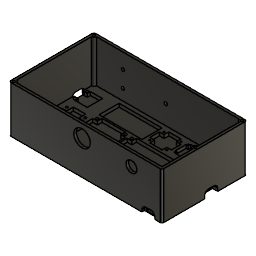
Base TestBenchV2 v1 (Autodesk Fusion 360 design; units mm, degrees)
part number: 2025-10-03-12-35-34-740
Autodesk Fusion 360 part; units mm, degrees
(part 1 of 3)
sketch "Boceto4" plane through (0, 0, 0) normal (0, 0, 1) x (1, 0, 0)
  line L0 (165, 0) -> (165, 100)
  line L1 (165, 0) -> (0, 0)
  line L2 (165, 100) -> (0, 100)
  line L3 (0, 100) -> (0, 0)
  line L4 (0, 100) -> (-15, 100)
  line L5 (-15, 100) -> (-15, 0)
  line L6 (-15, 0) -> (0, 0)
  line L7 (0, 0) -> (0, 100)
  dimension "d157" = 165
  dimension "d168" = 100
  dimension "d277" = 15
  constraint vertical L0
  constraint perpendicular L0 L1
  constraint perpendicular L0 L2
  constraint coincident L1.end L3.end
  constraint horizontal L4
  constraint vertical L5
  constraint horizontal L6
  constraint vertical L7
  constraint collinear L1 L6
  measures "d157" distance of L0.start L1.end
  measures "d168" distance of L1 L2
  measures "d277" distance of L2.end L4.end
extrude "Extruir2" add sketch "Boceto4" along normal blind 5
sketch "Boceto1" plane through (0, 0, 5) normal (0, 0, 1) x (1, 0, 0)
  line L0 (22, 67) -> (60.5, 67)
  line L1 (60.5, 67) -> (60.5, 16.5)
  line L2 (60.5, 16.5) -> (22, 16.5)
  line L3 (22, 16.5) -> (22, 67)
  line L4 (62.5, 67) -> (137.5, 67)
  line L5 (137.5, 67) -> (137.5, 16.5)
  line L6 (137.5, 16.5) -> (62.5, 16.5)
  line L7 (62.5, 16.5) -> (62.5, 67)
  line L8 (103.5, 92.5293) -> (147, 92.5293)
  line L9 (147, 74.5293) -> (103.5, 74.5293)
  line L10 (103.5, 74.5293) -> (103.5, 92.5293)
  line L11 (75, 92.5) -> (100.5, 92.5)
  line L12 (100.5, 92.5) -> (100.5, 70.2)
  line L13 (100.5, 70.2) -> (75, 70.2)
  line L14 (75, 70.2) -> (75, 92.5)
  line L15 (165, 0) -> (165, 100)
  line L16 (165, 100) -> (-15, 100)
  line L17 (-15, 0) -> (165, 0)
  line L18 (22, 92.5) -> (72.5, 92.5)
  line L19 (72.5, 92.5) -> (72.5, 69)
  line L20 (72.5, 69) -> (22, 69)
  line L21 (22, 69) -> (22, 92.5)
  line L22 (-10.5, 87.487) -> (7.5, 87.487)
  line L23 (7.5, 87.487) -> (7.5, 69.487)
  line L24 (7.5, 69.487) -> (-10.5, 69.487)
  line L25 (-7.0254, 61.685) -> (19.3746, 61.685)
  line L26 (19.3746, 61.685) -> (19.3746, 24.785)
  line L27 (19.3746, 24.785) -> (-7.0254, 24.785)
  line L28 (-7.0254, 24.785) -> (-7.0254, 61.685)
  line L29 (139.5, 49) -> (139.5, 67)
  line L30 (157.5, 49) -> (139.5, 49)
  line L31 (139.5, 67) -> (157.5, 67)
  line L32 (140, 4.5) -> (140, 22.5)
  line L33 (140, 22.5) -> (158, 22.5)
  line L34 (158, 22.5) -> (158, 4.5)
  line L35 (-10.5, 73.487) -> (-12, 73.487)
  line L36 (-12, 83.487) -> (-12, 73.487)
  line L37 (-10.5, 69.487) -> (-10.5, 73.487)
  line L38 (-10.5, 83.487) -> (-10.5, 87.487)
  line L39 (144, 3) -> (144, 4.5)
  line L40 (154, 3) -> (154, 4.5)
  line L41 (158, 4.5) -> (154, 4.5)
  line L42 (144, 4.5) -> (140, 4.5)
  line L43 (159, 63) -> (157.5, 63)
  line L44 (157.5, 53) -> (159, 53)
  line L45 (165, 63) -> (165, 53)
  line L46 (157.5, 67) -> (157.5, 63)
  line L47 (157.5, 53) -> (157.5, 49)
  circle A0 centre (-12, 97) radius 1.5
  circle A1 centre (162, 97) radius 1.5
  circle A2 centre (-12, 3) radius 1.5
  circle A3 centre (162, 42) radius 1.5
  line L48 (147, 89.5293) -> (165, 89.5293)
  line L49 (147, 77.5293) -> (165, 77.5293)
  line L50 (147, 92.5293) -> (147, 89.5293)
  line L51 (147, 77.5293) -> (147, 74.5293)
  line L52 (165, 89.5293) -> (165, 77.5293)
  line L53 (112.793, 73.7793) -> (132.793, 73.7793)
  line L54 (132.793, 73.7793) -> (132.793, 67.7793)
  line L55 (132.793, 67.7793) -> (112.793, 67.7793)
  line L56 (112.793, 67.7793) -> (112.793, 73.7793)
  line L57 (-15, 100) -> (-15, 0)
  line L58 (154, 3) -> (144, 3)
  line L59 (-12, 83.487) -> (-10.5, 83.487)
  line L60 (159, 63) -> (159, 53)
  dimension "d7" = 38.5
  dimension "d8" = 50.5
  dimension "d9" = 75
  dimension "d10" = 50.5
  dimension "d17" = 43.5
  dimension "d18" = 18
  dimension "d21" = 25.5
  dimension "d22" = 22.3
  dimension "d160" = 50.5
  dimension "d161" = 23.5
  dimension "d162" = 18
  dimension "d163" = 18
  dimension "d164" = 26.4
  dimension "d165" = 36.9
  dimension "d169" = 18
  dimension "d170" = 18
  dimension "d171" = 18
  dimension "d172" = 18
  dimension "d174" = 4
  dimension "d175" = 4
  dimension "d176" = 4
  dimension "d177" = 4
  dimension "d179" = 4
  dimension "d180" = 3
  dimension "d181" = 3
  dimension "d183" = 3
  dimension "d184" = 3
  dimension "d185" = 3
  dimension "d186" = 3
  dimension "d187" = 3
  dimension "d189" = 3
  dimension "d190" = 3
  dimension "d191" = 7
  dimension "d194" = 3
  dimension "d195" = 3
  dimension "d266" = 20
  dimension "d267" = 6
  dimension "d268" = 0.75
  dimension "d278" = 3
  dimension "d279" = 3
  dimension "d280" = 1.5
  dimension "d310" = 3
  dimension "d311" = 1.5
  dimension "d312" = 3
  dimension "d313" = 1.5
  constraint horizontal L0
  constraint vertical L1
  constraint horizontal L2
  constraint vertical L3
  constraint horizontal L4
  constraint vertical L5
  constraint horizontal L6
  constraint vertical L7
  constraint horizontal L8
  constraint vertical L50
  constraint horizontal L9
  constraint vertical L10
  constraint horizontal L11
  constraint vertical L12
  constraint horizontal L13
  constraint vertical L14
  constraint horizontal L18
  constraint vertical L19
  constraint horizontal L20
  constraint vertical L21
  constraint horizontal L22
  constraint vertical L23
  constraint horizontal L24
  constraint vertical L37
  constraint horizontal L25
  constraint vertical L26
  constraint horizontal L27
  constraint vertical L28
  constraint horizontal L31
  constraint vertical L46
  constraint horizontal L30
  constraint vertical L29
  constraint horizontal L33
  constraint vertical L34
  constraint horizontal L41
  constraint vertical L32
  constraint coincident L38.start L37
  constraint collinear L37 L38
  constraint coincident L39.end L41
  constraint perpendicular L39 L41
  constraint perpendicular L40 L41
  constraint collinear L41 L42
  constraint coincident L15 L45.start
  constraint perpendicular L43 L46
  constraint coincident L44.start L46
  constraint coincident L15 L45.end
  constraint perpendicular L15 L44
  constraint collinear L46 L47
  constraint coincident L15 L48.end
  constraint perpendicular L15 L48
  constraint coincident L49.start L50
  constraint coincident L15 L49.end
  constraint perpendicular L15 L49
  constraint collinear L50 L51
  constraint horizontal L53
  constraint vertical L54
  constraint horizontal L55
  constraint vertical L56
  constraint horizontal L58
  constraint perpendicular L38 L59
  constraint vertical L60
  measures "d7" distance of L0.start L0.end
  measures "d8" distance of L0.start L2.end
  measures "d9" distance of L4.start L4.end
  measures "d10" distance of L4.start L6.end
  measures "d17" distance of L8.start L8.end
  measures "d18" distance of L8.start L9.end
  measures "d21" distance of L11.start L11.end
  measures "d22" distance of L11.start L13.end
  measures "d160" distance of L18.start L18.end
  measures "d161" distance of L18.start L20.end
  measures "d162" distance of L22.start L22.end
  measures "d163" distance of L22.start L24.end
  measures "d164" distance of L25.start L25.end
  measures "d165" distance of L25.start L27.end
  measures "d169" distance of L31.end L29.end
  measures "d170" distance of L29.start L29.end
  measures "d171" distance of L32.end L33.end
  measures "d172" distance of L32.end L32.start
  measures "d174" distance of L24 L35
  measures "d175" distance of L34 L40
  measures "d176" distance of L32 L39
  measures "d177" distance of L31 L43
  measures "d179" distance of L30 L44
  measures "d180" diameter of A0
  measures "d181" distance of L16 A0.centre
  measures "d183" diameter of A1
  measures "d184" distance of L15 A1.centre
  measures "d185" distance of L16 A1.centre
  measures "d186" diameter of A2
  measures "d187" distance of L17 A2.centre
  measures "d189" diameter of A3
  measures "d190" distance of L15 A3.centre
  measures "d191" distance of L30 A3.centre
  measures "d194" distance of L8 L48
  measures "d195" distance of L9 L49
  measures "d266" distance of L53.start L53.end
  measures "d267" distance of L53.start L55.end
  measures "d268" distance of L9 L53
  measures "d278" horizontal distance of A2.centre L17.start
  measures "d279" distance of A0.centre L57
  measures "d280" distance of L36 L38
  measures "d310" distance of L36 L57
  measures "d311" distance of L40.start L40.end
  measures "d312" distance of L17 L58
  measures "d313" distance of L43.end L43.start
extrude "Extruir3" cut sketch "Boceto1" against normal blind 4 contours L0 L1 L2 L3 | L4 L5 L6 L7 | L8 L9 L10 L15 L48 L49 L50 L51 L52 | L11 L12 L13 L14 | L18 L19 L20 L21 | L22 L23 L24 L35 L36 L37 L38 L59 | L25 L26 L27 L28 | L29 L30 L31 L43 L44 L46 L47 L60 | L32 L33 L34 L39 L40 L41 L42 L58 | A0 | A1 | A2 | A3 | L53 L54 L55 L56
sketch "Boceto15" plane through (0, 0, 1) normal (0, 0, 1) x (-1, 0, 0)
  line L0 (-140.5294, -30.8793) -> (-140.5328, -29.1153)
  line L1 (-140.5328, -29.1153) -> (-140.2681, -29.1148)
  line L2 (-140.2681, -29.1148) -> (-140.2648, -30.8788)
  line L3 (-140.2648, -30.8788) -> (-139.6058, -30.8776)
  line L4 (-139.6058, -30.8776) -> (-139.6054, -31.1136)
  line L5 (-139.6054, -31.1136) -> (-141.1906, -31.1166)
  line L6 (-141.1906, -31.1166) -> (-141.1911, -30.8806)
  line L7 (-141.1911, -30.8806) -> (-140.5294, -30.8793)
  spline S0 degree 3 poles (-143.6617, -29.1663) (-143.604, -29.1955) (-143.4902, -29.2532) (-143.412, -29.3541) (-143.3734, -29.4038) knots 0 0 0 0 0.019136 0.037772 0.037772 0.037772 0.037772
  spline S1 degree 3 poles (-143.3734, -29.4038) (-143.3426, -29.4589) (-143.2802, -29.5708) (-143.2687, -29.6984) (-143.2629, -29.7631) knots 0 0 0 0 0.018713 0.037965 0.037965 0.037965 0.037965
  line L8 (-143.2629, -29.7631) -> (-143.5125, -29.7854)
  spline S2 degree 3 poles (-143.5125, -29.7854) (-143.5197, -29.7389) (-143.533, -29.6519) (-143.5757, -29.5751) (-143.5955, -29.5393) knots 0 0 0 0 0.013975 0.026155 0.026155 0.026155 0.026155
  spline S3 degree 3 poles (-143.5955, -29.5393) (-143.6215, -29.5083) (-143.6771, -29.4418) (-143.7554, -29.4042) (-143.797, -29.3842) knots 0 0 0 0 0.012002 0.025694 0.025694 0.025694 0.025694
  spline S4 degree 3 poles (-143.797, -29.3842) (-143.8449, -29.3669) (-143.9441, -29.3313) (-144.0496, -29.3274) (-144.1041, -29.3254) knots 0 0 0 0 0.015163 0.031432 0.031432 0.031432 0.031432
  spline S5 degree 3 poles (-144.1041, -29.3254) (-144.152, -29.327) (-144.2433, -29.3299) (-144.3302, -29.3577) (-144.3714, -29.3709) knots 0 0 0 0 0.014301 0.027232 0.027232 0.027232 0.027232
  spline S6 degree 3 poles (-144.3714, -29.3709) (-144.4068, -29.3864) (-144.4732, -29.4155) (-144.5213, -29.4695) (-144.5438, -29.4947) knots 0 0 0 0 0.011435 0.021444 0.021444 0.021444 0.021444
  spline S7 degree 3 poles (-144.5438, -29.4947) (-144.5602, -29.5213) (-144.5928, -29.5739) (-144.5977, -29.6356) (-144.6001, -29.666) knots 0 0 0 0 0.009237 0.018267 0.018267 0.018267 0.018267
  spline S8 degree 3 poles (-144.6001, -29.666) (-144.5979, -29.6962) (-144.5936, -29.7557) (-144.5611, -29.8057) (-144.5452, -29.8303) knots 0 0 0 0 0.008921 0.017573 0.017573 0.017573 0.017573
  spline S9 degree 3 poles (-144.5452, -29.8303) (-144.5221, -29.8534) (-144.4705, -29.9052) (-144.4025, -29.9327) (-144.3649, -29.948) knots 0 0 0 0 0.009698 0.021725 0.021725 0.021725 0.021725
  spline S10 degree 3 poles (-144.3649, -29.948) (-144.3219, -29.9617) (-144.2045, -29.9991) (-144.0846, -30.0271) (-144.0086, -30.0449) knots 0 0 0 0 0.013533 0.036931 0.036931 0.036931 0.036931
  spline S11 degree 3 poles (-144.0086, -30.0449) (-143.9296, -30.0636) (-143.7975, -30.0949) (-143.6725, -30.1477) (-143.6223, -30.169) knots 0 0 0 0 0.024297 0.040637 0.040637 0.040637 0.040637
  spline S12 degree 3 poles (-143.6223, -30.169) (-143.5783, -30.1943) (-143.4947, -30.2423) (-143.4361, -30.3187) (-143.4084, -30.3548) knots 0 0 0 0 0.015064 0.02858 0.02858 0.02858 0.02858
  spline S13 degree 3 poles (-143.4084, -30.3548) (-143.3879, -30.3932) (-143.3462, -30.471) (-143.3406, -30.559) (-143.3377, -30.6036) knots 0 0 0 0 0.012908 0.026139 0.026139 0.026139 0.026139
  spline S14 degree 3 poles (-143.3377, -30.6036) (-143.3413, -30.6535) (-143.3487, -30.7542) (-143.3981, -30.8424) (-143.4231, -30.8869) knots 0 0 0 0 0.014805 0.02991 0.02991 0.02991 0.02991
  spline S15 degree 3 poles (-143.4231, -30.8869) (-143.4559, -30.9285) (-143.5237, -31.0148) (-143.6226, -31.0625) (-143.6738, -31.0872) knots 0 0 0 0 0.01568 0.032466 0.032466 0.032466 0.032466
  spline S16 degree 3 poles (-143.6738, -31.0872) (-143.7313, -31.1072) (-143.8501, -31.1485) (-143.9758, -31.1535) (-144.0406, -31.1561) knots 0 0 0 0 0.018164 0.037509 0.037509 0.037509 0.037509
  spline S17 degree 3 poles (-144.0406, -31.1561) (-144.111, -31.1539) (-144.2454, -31.1496) (-144.3725, -31.106) (-144.433, -31.0852) knots 0 0 0 0 0.021001 0.040071 0.040071 0.040071 0.040071
  spline S18 degree 3 poles (-144.433, -31.0852) (-144.4859, -31.0593) (-144.589, -31.0088) (-144.6601, -30.9188) (-144.6946, -30.8749) knots 0 0 0 0 0.017437 0.033952 0.033952 0.033952 0.033952
  spline S19 degree 3 poles (-144.6946, -30.8749) (-144.7217, -30.8267) (-144.7766, -30.7286) (-144.7878, -30.6168) (-144.7935, -30.56) knots 0 0 0 0 0.016416 0.033327 0.033327 0.033327 0.033327
  line L9 (-144.7935, -30.56) -> (-144.5397, -30.5404)
  spline S20 degree 3 poles (-144.5397, -30.5404) (-144.5301, -30.5986) (-144.5119, -30.7081) (-144.4362, -30.7888) (-144.4007, -30.8266) knots 0 0 0 0 0.017238 0.032462 0.032462 0.032462 0.032462
  spline S21 degree 3 poles (-144.4007, -30.8266) (-144.3531, -30.8547) (-144.2461, -30.9179) (-144.1213, -30.9211) (-144.052, -30.9228) knots 0 0 0 0 0.016321 0.036707 0.036707 0.036707 0.036707
  spline S22 degree 3 poles (-144.052, -30.9228) (-143.9811, -30.9216) (-143.8568, -30.9195) (-143.7486, -30.8598) (-143.7022, -30.8342) knots 0 0 0 0 0.02087 0.036564 0.036564 0.036564 0.036564
  spline S23 degree 3 poles (-143.7022, -30.8342) (-143.6702, -30.8041) (-143.6086, -30.746) (-143.5979, -30.6622) (-143.5928, -30.6218) knots 0 0 0 0 0.012728 0.024562 0.024562 0.024562 0.024562
  spline S24 degree 3 poles (-143.5928, -30.6218) (-143.596, -30.5876) (-143.6023, -30.5198) (-143.6482, -30.4695) (-143.6709, -30.4446) knots 0 0 0 0 0.010013 0.019843 0.019843 0.019843 0.019843
  spline S25 degree 3 poles (-143.6709, -30.4446) (-143.7162, -30.4195) (-143.8409, -30.3503) (-143.981, -30.3213) (-144.0702, -30.3028) knots 0 0 0 0 0.01549 0.042576 0.042576 0.042576 0.042576
  spline S26 degree 3 poles (-144.0702, -30.3028) (-144.1616, -30.2826) (-144.3119, -30.2493) (-144.4565, -30.1967) (-144.5131, -30.1761) knots 0 0 0 0 0.028046 0.046113 0.046113 0.046113 0.046113
  spline S27 degree 3 poles (-144.5131, -30.1761) (-144.5665, -30.1491) (-144.6665, -30.0986) (-144.738, -30.0127) (-144.7714, -29.9726) knots 0 0 0 0 0.017709 0.033187 0.033187 0.033187 0.033187
  spline S28 degree 3 poles (-144.7714, -29.9726) (-144.7957, -29.9294) (-144.8455, -29.8412) (-144.8519, -29.74) (-144.8551, -29.6883) knots 0 0 0 0 0.014678 0.02998 0.02998 0.02998 0.02998
  spline S29 degree 3 poles (-144.8551, -29.6883) (-144.8512, -29.6356) (-144.8433, -29.5286) (-144.7909, -29.4349) (-144.7643, -29.3874) knots 0 0 0 0 0.015669 0.031781 0.031781 0.031781 0.031781
  spline S30 degree 3 poles (-144.7643, -29.3874) (-144.7298, -29.3425) (-144.6586, -29.2499) (-144.5553, -29.1953) (-144.5021, -29.1672) knots 0 0 0 0 0.016779 0.034595 0.034595 0.034595 0.034595
  spline S31 degree 3 poles (-144.5021, -29.1672) (-144.4422, -29.1442) (-144.3182, -29.0967) (-144.1854, -29.091) (-144.1168, -29.088) knots 0 0 0 0 0.019123 0.039562 0.039562 0.039562 0.039562
  spline S32 degree 3 poles (-144.1168, -29.088) (-144.0329, -29.09) (-143.8771, -29.0937) (-143.7297, -29.1434) (-143.6617, -29.1663) knots 0 0 0 0 0.025027 0.046416 0.046416 0.046416 0.046416
  spline S33 degree 3 poles (-148.0234, -29.163) (-147.9747, -29.1532) (-147.8683, -29.1317) (-147.7597, -29.1299) (-147.7008, -29.1289) knots 0 0 0 0 0.014862 0.032497 0.032497 0.032497 0.032497
  line L10 (-147.7008, -29.1289) -> (-146.9382, -29.1275)
  line L11 (-146.9382, -29.1275) -> (-146.9344, -31.1275)
  line L12 (-146.9344, -31.1275) -> (-147.6847, -31.1289)
  spline S34 degree 3 poles (-147.6847, -31.1289) (-147.7542, -31.1278) (-147.8799, -31.1257) (-147.9992, -31.0865) (-148.0525, -31.0689) knots 0 0 0 0 0.020707 0.037453 0.037453 0.037453 0.037453
  spline S35 degree 3 poles (-148.0525, -31.0689) (-148.0961, -31.0461) (-148.183, -31.0008) (-148.2409, -30.9217) (-148.2698, -30.8824) knots 0 0 0 0 0.014555 0.028975 0.028975 0.028975 0.028975
  spline S36 degree 3 poles (-148.2698, -30.8824) (-148.2927, -30.8404) (-148.3377, -30.758) (-148.3451, -30.6644) (-148.3487, -30.6186) knots 0 0 0 0 0.014187 0.027818 0.027818 0.027818 0.027818
  spline S37 degree 3 poles (-148.3487, -30.6186) (-148.3458, -30.5763) (-148.3399, -30.4909) (-148.2998, -30.4152) (-148.2796, -30.377) knots 0 0 0 0 0.01257 0.025379 0.025379 0.025379 0.025379
  spline S38 degree 3 poles (-148.2796, -30.377) (-148.2526, -30.3405) (-148.196, -30.2643) (-148.1131, -30.218) (-148.0698, -30.1938) knots 0 0 0 0 0.013451 0.028132 0.028132 0.028132 0.028132
  spline S39 degree 3 poles (-148.0698, -30.1938) (-148.1261, -30.174) (-148.2339, -30.1361) (-148.3119, -30.0527) (-148.3492, -30.0129) knots 0 0 0 0 0.017587 0.033722 0.033722 0.033722 0.033722
  spline S40 degree 3 poles (-148.3492, -30.0129) (-148.3777, -29.9676) (-148.436, -29.8751) (-148.4435, -29.766) (-148.4473, -29.7102) knots 0 0 0 0 0.015782 0.032266 0.032266 0.032266 0.032266
  spline S41 degree 3 poles (-148.4473, -29.7102) (-148.445, -29.6644) (-148.4405, -29.5738) (-148.4057, -29.4902) (-148.3884, -29.4488) knots 0 0 0 0 0.013638 0.026971 0.026971 0.026971 0.026971
  spline S42 degree 3 poles (-148.3884, -29.4488) (-148.3684, -29.4115) (-148.3305, -29.3407) (-148.2705, -29.2875) (-148.2421, -29.2623) knots 0 0 0 0 0.012583 0.02387 0.02387 0.02387 0.02387
  spline S43 degree 3 poles (-148.2421, -29.2623) (-148.2101, -29.2415) (-148.1423, -29.1974) (-148.0645, -29.1749) (-148.0234, -29.163) knots 0 0 0 0 0.011395 0.024144 0.024144 0.024144 0.024144
  line L13 (-150.9489, -30.7067) -> (-150.9519, -29.1351)
  line L14 (-150.9519, -29.1351) -> (-150.6982, -29.1346)
  line L15 (-150.6982, -29.1346) -> (-150.6944, -31.1346)
  line L16 (-150.6944, -31.1346) -> (-150.9659, -31.1352)
  line L17 (-150.9659, -31.1352) -> (-152.0193, -29.5669)
  line L18 (-152.0193, -29.5669) -> (-152.0163, -31.1371)
  line L19 (-152.0163, -31.1371) -> (-152.2701, -31.1376)
  line L20 (-152.2701, -31.1376) -> (-152.2739, -29.1376)
  line L21 (-152.2739, -29.1376) -> (-152.0024, -29.1371)
  line L22 (-152.0024, -29.1371) -> (-150.9489, -30.7067)
  line L23 (-155.0321, -30.0856) -> (-155.0339, -29.1429)
  line L24 (-155.0339, -29.1429) -> (-154.7692, -29.1424)
  line L25 (-154.7692, -29.1424) -> (-154.7654, -31.1424)
  line L26 (-154.7654, -31.1424) -> (-155.0301, -31.1429)
  line L27 (-155.0301, -31.1429) -> (-155.0316, -30.3216)
  line L28 (-155.0316, -30.3216) -> (-156.0712, -30.3236)
  line L29 (-156.0712, -30.3236) -> (-156.0696, -31.1448)
  line L30 (-156.0696, -31.1448) -> (-156.3343, -31.1453)
  line L31 (-156.3343, -31.1453) -> (-156.3381, -29.1453)
  line L32 (-156.3381, -29.1453) -> (-156.0734, -29.1448)
  line L33 (-156.0734, -29.1448) -> (-156.0716, -30.0875)
  line L34 (-156.0716, -30.0875) -> (-155.0321, -30.0856)
  line L35 (-143.2927, -26.2352) -> (-143.2932, -25.9992)
  line L36 (-143.2932, -25.9992) -> (-141.8007, -25.9963)
  line L37 (-141.8007, -25.9963) -> (-141.7969, -27.9963)
  line L38 (-141.7969, -27.9963) -> (-143.243, -27.9991)
  line L39 (-143.243, -27.9991) -> (-143.2435, -27.763)
  line L40 (-143.2435, -27.763) -> (-142.062, -27.7608)
  line L41 (-142.062, -27.7608) -> (-142.0632, -27.1483)
  line L42 (-142.0632, -27.1483) -> (-143.1696, -27.1504)
  line L43 (-143.1696, -27.1504) -> (-143.17, -26.9157)
  line L44 (-143.17, -26.9157) -> (-142.0636, -26.9136)
  line L45 (-142.0636, -26.9136) -> (-142.0649, -26.2328)
  line L46 (-142.0649, -26.2328) -> (-143.2927, -26.2352)
  spline S44 degree 3 poles (-145.7899, -25.9698) (-145.6994, -25.9773) (-145.5229, -25.9921) (-145.3967, -26.1159) (-145.3353, -26.1763) knots 0 0 0 0 0.026334 0.051363 0.051363 0.051363 0.051363
  spline S45 degree 3 poles (-145.3353, -26.1763) (-145.2777, -26.2834) (-145.1422, -26.5356) (-145.1382, -26.8234) (-145.1359, -26.989) knots 0 0 0 0 0.036009 0.08476 0.08476 0.08476 0.08476
  spline S46 degree 3 poles (-145.1359, -26.989) (-145.1371, -27.0963) (-145.1394, -27.2896) (-145.1867, -27.4768) (-145.2078, -27.5601) knots 0 0 0 0 0.032061 0.057736 0.057736 0.057736 0.057736
  spline S47 degree 3 poles (-145.2078, -27.5601) (-145.2335, -27.6269) (-145.2823, -27.7536) (-145.3786, -27.849) (-145.4241, -27.8941) knots 0 0 0 0 0.021191 0.040192 0.040192 0.040192 0.040192
  spline S48 degree 3 poles (-145.4241, -27.8941) (-145.4766, -27.9284) (-145.5864, -28.0001) (-145.7176, -28.008) (-145.7861, -28.0121) knots 0 0 0 0 0.018481 0.038665 0.038665 0.038665 0.038665
  spline S49 degree 3 poles (-145.7861, -28.0121) (-145.8372, -28.0099) (-145.9354, -28.0058) (-146.0254, -27.9666) (-146.0686, -27.9478) knots 0 0 0 0 0.015196 0.029197 0.029197 0.029197 0.029197
  spline S50 degree 3 poles (-146.0686, -27.9478) (-146.1075, -27.9236) (-146.1866, -27.8745) (-146.2416, -27.7994) (-146.2695, -27.7613) knots 0 0 0 0 0.013619 0.027641 0.027641 0.027641 0.027641
  spline S51 degree 3 poles (-146.2695, -27.7613) (-146.2949, -27.717) (-146.3487, -27.6231) (-146.3785, -27.519) (-146.3942, -27.4641) knots 0 0 0 0 0.01527 0.032333 0.032333 0.032333 0.032333
  spline S52 degree 3 poles (-146.3942, -27.4641) (-146.4074, -27.3957) (-146.4375, -27.2397) (-146.4392, -27.0808) (-146.4401, -26.9915) knots 0 0 0 0 0.020858 0.04757 0.04757 0.04757 0.04757
  spline S53 degree 3 poles (-146.4401, -26.9915) (-146.4389, -26.8849) (-146.4366, -26.6925) (-146.3898, -26.5062) (-146.3689, -26.4231) knots 0 0 0 0 0.031856 0.057454 0.057454 0.057454 0.057454
  spline S54 degree 3 poles (-146.3689, -26.4231) (-146.3434, -26.3563) (-146.2949, -26.2294) (-146.1988, -26.1338) (-146.1533, -26.0885) knots 0 0 0 0 0.021185 0.040213 0.040213 0.040213 0.040213
  spline S55 degree 3 poles (-146.1533, -26.0885) (-146.1007, -26.054) (-145.9906, -25.9817) (-145.8588, -25.9739) (-145.7899, -25.9698) knots 0 0 0 0 0.018535 0.038823 0.038823 0.038823 0.038823
  spline S56 degree 3 poles (-156.2493, -22.8696) (-156.1642, -22.8718) (-156.0105, -22.8759) (-155.8778, -22.9521) (-155.8186, -22.9861) knots 0 0 0 0 0.025053 0.045234 0.045234 0.045234 0.045234
  spline S57 degree 3 poles (-155.8186, -22.9861) (-155.7733, -23.0319) (-155.6771, -23.1292) (-155.6457, -23.2629) (-155.629, -23.3336) knots 0 0 0 0 0.01895 0.040278 0.040278 0.040278 0.040278
  line L47 (-155.629, -23.3336) -> (-155.8718, -23.3723)
  spline S58 degree 3 poles (-155.8718, -23.3723) (-155.8808, -23.3273) (-155.898, -23.2418) (-155.9578, -23.1787) (-155.9861, -23.1488) knots 0 0 0 0 0.013461 0.025563 0.025563 0.025563 0.025563
  spline S59 degree 3 poles (-155.9861, -23.1488) (-156.0225, -23.1262) (-156.1022, -23.0767) (-156.1964, -23.0733) (-156.2475, -23.0715) knots 0 0 0 0 0.012631 0.027679 0.027679 0.027679 0.027679
  spline S60 degree 3 poles (-156.2475, -23.0715) (-156.298, -23.0728) (-156.3879, -23.075) (-156.4647, -23.1208) (-156.4984, -23.1409) knots 0 0 0 0 0.014834 0.026419 0.026419 0.026419 0.026419
  spline S61 degree 3 poles (-156.4984, -23.1409) (-156.5222, -23.1642) (-156.568, -23.209) (-156.5761, -23.2723) (-156.58, -23.3027) knots 0 0 0 0 0.009682 0.0186 0.0186 0.0186 0.0186
  spline S62 degree 3 poles (-156.58, -23.3027) (-156.5768, -23.329) (-156.5703, -23.3824) (-156.5285, -23.4163) (-156.5074, -23.4335) knots 0 0 0 0 0.007652 0.015492 0.015492 0.015492 0.015492
  spline S63 degree 3 poles (-156.5074, -23.4335) (-156.4783, -23.4465) (-156.3975, -23.4826) (-156.3113, -23.5031) (-156.2562, -23.5163) knots 0 0 0 0 0.009553 0.026493 0.026493 0.026493 0.026493
  spline S64 degree 3 poles (-156.2562, -23.5163) (-156.1793, -23.5354) (-156.052, -23.567) (-155.9299, -23.6147) (-155.8815, -23.6336) knots 0 0 0 0 0.023737 0.039299 0.039299 0.039299 0.039299
  spline S65 degree 3 poles (-155.8815, -23.6336) (-155.8491, -23.6512) (-155.7862, -23.6855) (-155.7436, -23.7431) (-155.723, -23.771) knots 0 0 0 0 0.010927 0.021211 0.021211 0.021211 0.021211
  spline S66 degree 3 poles (-155.723, -23.771) (-155.7072, -23.8013) (-155.6754, -23.8622) (-155.671, -23.9308) (-155.6688, -23.9654) knots 0 0 0 0 0.010103 0.020373 0.020373 0.020373 0.020373
  spline S67 degree 3 poles (-155.6688, -23.9654) (-155.6705, -23.9969) (-155.6739, -24.0595) (-155.6999, -24.1166) (-155.7127, -24.1448) knots 0 0 0 0 0.009394 0.018625 0.018625 0.018625 0.018625
  spline S68 degree 3 poles (-155.7127, -24.1448) (-155.7288, -24.1712) (-155.761, -24.224) (-155.8091, -24.2628) (-155.8332, -24.2822) knots 0 0 0 0 0.009191 0.018393 0.018393 0.018393 0.018393
  spline S69 degree 3 poles (-155.8332, -24.2822) (-155.8553, -24.2961) (-155.9041, -24.327) (-155.9592, -24.3445) (-155.9893, -24.3541) knots 0 0 0 0 0.007816 0.017247 0.017247 0.017247 0.017247
  spline S70 degree 3 poles (-155.9893, -24.3541) (-156.0233, -24.3627) (-156.0929, -24.3804) (-156.1646, -24.3827) (-156.2014, -24.3838) knots 0 0 0 0 0.010482 0.021472 0.021472 0.021472 0.021472
  spline S71 degree 3 poles (-156.2014, -24.3838) (-156.2552, -24.3824) (-156.3573, -24.3796) (-156.4548, -24.3495) (-156.5009, -24.3353) knots 0 0 0 0 0.01606 0.030471 0.030471 0.030471 0.030471
  spline S72 degree 3 poles (-156.5009, -24.3353) (-156.5402, -24.3187) (-156.6133, -24.2879) (-156.6668, -24.2296) (-156.6915, -24.2026) knots 0 0 0 0 0.012608 0.023462 0.023462 0.023462 0.023462
  spline S73 degree 3 poles (-156.6915, -24.2026) (-156.7107, -24.1707) (-156.7524, -24.1012) (-156.7681, -24.0215) (-156.7765, -23.9784) knots 0 0 0 0 0.011092 0.024145 0.024145 0.024145 0.024145
  line L48 (-156.7765, -23.9784) -> (-156.5365, -23.9452)
  spline S74 degree 3 poles (-156.5365, -23.9452) (-156.5288, -23.98) (-156.514, -24.0475) (-156.465, -24.0961) (-156.4413, -24.1196) knots 0 0 0 0 0.010457 0.02025 0.02025 0.02025 0.02025
  spline S75 degree 3 poles (-156.4413, -24.1196) (-156.4105, -24.1378) (-156.3424, -24.1781) (-156.263, -24.1806) (-156.2195, -24.1819) knots 0 0 0 0 0.01057 0.023371 0.023371 0.023371 0.023371
  spline S76 degree 3 poles (-156.2195, -24.1819) (-156.1701, -24.1815) (-156.0849, -24.1806) (-156.0097, -24.1418) (-155.9781, -24.1256) knots 0 0 0 0 0.014563 0.025087 0.025087 0.025087 0.025087
  spline S77 degree 3 poles (-155.9781, -24.1256) (-155.9571, -24.1069) (-155.9173, -24.0716) (-155.9097, -24.0191) (-155.9061, -23.9945) knots 0 0 0 0 0.00814 0.015395 0.015395 0.015395 0.015395
  spline S78 degree 3 poles (-155.9061, -23.9945) (-155.9074, -23.9789) (-155.91, -23.9477) (-155.9275, -23.9216) (-155.9363, -23.9086) knots 0 0 0 0 0.004598 0.009239 0.009239 0.009239 0.009239
  spline S79 degree 3 poles (-155.9363, -23.9086) (-155.9485, -23.8957) (-155.9753, -23.8674) (-156.0111, -23.8518) (-156.0305, -23.8433) knots 0 0 0 0 0.005284 0.01157 0.01157 0.01157 0.01157
  spline S80 degree 3 poles (-156.0305, -23.8433) (-156.0547, -23.8357) (-156.1266, -23.8132) (-156.1993, -23.7938) (-156.2475, -23.7809) knots 0 0 0 0 0.007605 0.022583 0.022583 0.022583 0.022583
  spline S81 degree 3 poles (-156.2475, -23.7809) (-156.3218, -23.7614) (-156.4447, -23.7289) (-156.564, -23.6851) (-156.6113, -23.6677) knots 0 0 0 0 0.023005 0.038119 0.038119 0.038119 0.038119
  spline S82 degree 3 poles (-156.6113, -23.6677) (-156.6436, -23.6516) (-156.7068, -23.6202) (-156.7514, -23.5657) (-156.7732, -23.5391) knots 0 0 0 0 0.010681 0.020888 0.020888 0.020888 0.020888
  spline S83 degree 3 poles (-156.7732, -23.5391) (-156.7904, -23.5082) (-156.8266, -23.443) (-156.8304, -23.3684) (-156.8323, -23.3291) knots 0 0 0 0 0.010453 0.022074 0.022074 0.022074 0.022074
  spline S84 degree 3 poles (-156.8323, -23.3291) (-156.8292, -23.2885) (-156.823, -23.206) (-156.7819, -23.1342) (-156.7611, -23.0977) knots 0 0 0 0 0.012054 0.024479 0.024479 0.024479 0.024479
  spline S85 degree 3 poles (-156.7611, -23.0977) (-156.734, -23.0632) (-156.6777, -22.9919) (-156.5967, -22.9508) (-156.5548, -22.9295) knots 0 0 0 0 0.013001 0.026908 0.026908 0.026908 0.026908
  spline S86 degree 3 poles (-156.5548, -22.9295) (-156.5073, -22.9121) (-156.4087, -22.876) (-156.3037, -22.8718) (-156.2493, -22.8696) knots 0 0 0 0 0.015065 0.0313 0.0313 0.0313 0.0313
  spline S87 degree 3 poles (-140.6125, -23.065) (-140.683, -23.0698) (-140.8201, -23.0793) (-140.9336, -23.1565) (-140.9888, -23.194) knots 0 0 0 0 0.020781 0.040419 0.040419 0.040419 0.040419
  spline S88 degree 3 poles (-140.9888, -23.194) (-141.0364, -23.2445) (-141.1387, -23.353) (-141.1766, -23.4977) (-141.1968, -23.575) knots 0 0 0 0 0.020513 0.044031 0.044031 0.044031 0.044031
  line L49 (-141.1968, -23.575) -> (-141.4616, -23.5086)
  spline S89 degree 3 poles (-141.4616, -23.5086) (-141.4306, -23.4081) (-141.3718, -23.2172) (-141.2301, -23.0771) (-141.1631, -23.0108) knots 0 0 0 0 0.031006 0.058853 0.058853 0.058853 0.058853
  spline S90 degree 3 poles (-141.1631, -23.0108) (-141.0854, -22.9607) (-140.9247, -22.8571) (-140.7335, -22.8449) (-140.6347, -22.8386) knots 0 0 0 0 0.027244 0.056397 0.056397 0.056397 0.056397
  spline S91 degree 3 poles (-140.6347, -22.8386) (-140.5351, -22.842) (-140.35, -22.8483) (-140.1848, -22.931) (-140.1086, -22.9692) knots 0 0 0 0 0.029499 0.054784 0.054784 0.054784 0.054784
  spline S92 degree 3 poles (-140.1086, -22.9692) (-140.0445, -23.0191) (-139.9122, -23.1221) (-139.8379, -23.2724) (-139.7995, -23.35) knots 0 0 0 0 0.024039 0.049604 0.049604 0.049604 0.049604
  spline S93 degree 3 poles (-139.7995, -23.35) (-139.7685, -23.4353) (-139.7056, -23.6085) (-139.6971, -23.7926) (-139.6928, -23.8859) knots 0 0 0 0 0.027074 0.054928 0.054928 0.054928 0.054928
  spline S94 degree 3 poles (-139.6928, -23.8859) (-139.6966, -23.9847) (-139.7038, -24.1737) (-139.7765, -24.348) (-139.8111, -24.4311) knots 0 0 0 0 0.029398 0.056194 0.056194 0.056194 0.056194
  spline S95 degree 3 poles (-139.8111, -24.4311) (-139.8546, -24.5039) (-139.9406, -24.6478) (-140.0808, -24.7397) (-140.1501, -24.7851) knots 0 0 0 0 0.025058 0.049588 0.049588 0.049588 0.049588
  spline S96 degree 3 poles (-140.1501, -24.7851) (-140.2259, -24.8205) (-140.3797, -24.8922) (-140.5491, -24.9019) (-140.6349, -24.9068) knots 0 0 0 0 0.02485 0.050387 0.050387 0.050387 0.050387
  spline S97 degree 3 poles (-140.6349, -24.9068) (-140.7293, -24.9018) (-140.9104, -24.8922) (-141.0657, -24.7994) (-141.14, -24.755) knots 0 0 0 0 0.027889 0.053453 0.053453 0.053453 0.053453
  spline S98 degree 3 poles (-141.14, -24.755) (-141.2035, -24.6975) (-141.3349, -24.5788) (-141.3949, -24.4119) (-141.4259, -24.3258) knots 0 0 0 0 0.025285 0.052286 0.052286 0.052286 0.052286
  line L50 (-141.4259, -24.3258) -> (-141.1655, -24.2639)
  spline S99 degree 3 poles (-141.1655, -24.2639) (-141.1417, -24.3299) (-141.0981, -24.4514) (-141.0053, -24.5406) (-140.9629, -24.5814) knots 0 0 0 0 0.020699 0.03811 0.03811 0.03811 0.03811
  spline S100 degree 3 poles (-140.9629, -24.5814) (-140.9144, -24.6103) (-140.8119, -24.6713) (-140.6926, -24.6772) (-140.6299, -24.6803) knots 0 0 0 0 0.016702 0.035219 0.035219 0.035219 0.035219
  spline S101 degree 3 poles (-140.6299, -24.6803) (-140.5577, -24.6766) (-140.4203, -24.6695) (-140.3012, -24.6014) (-140.2447, -24.5691) knots 0 0 0 0 0.021343 0.040595 0.040595 0.040595 0.040595
  spline S102 degree 3 poles (-140.2447, -24.5691) (-140.1969, -24.5287) (-140.1005, -24.4473) (-140.0521, -24.3307) (-140.0276, -24.2719) knots 0 0 0 0 0.018474 0.037274 0.037274 0.037274 0.037274
  spline S103 degree 3 poles (-140.0276, -24.2719) (-140.0095, -24.2093) (-139.973, -24.0838) (-139.9681, -23.9532) (-139.9656, -23.8878) knots 0 0 0 0 0.019489 0.039044 0.039044 0.039044 0.039044
  spline S104 degree 3 poles (-139.9656, -23.8878) (-139.9681, -23.8075) (-139.9728, -23.6555) (-140.019, -23.5108) (-140.0408, -23.4425) knots 0 0 0 0 0.023964 0.045355 0.045355 0.045355 0.045355
  spline S105 degree 3 poles (-140.0408, -23.4425) (-140.0683, -23.3836) (-140.1218, -23.2693) (-140.2233, -23.1947) (-140.2726, -23.1585) knots 0 0 0 0 0.019149 0.037185 0.037185 0.037185 0.037185
  spline S106 degree 3 poles (-140.2726, -23.1585) (-140.326, -23.1311) (-140.4328, -23.0764) (-140.5526, -23.0688) (-140.6125, -23.065) knots 0 0 0 0 0.017797 0.035587 0.035587 0.035587 0.035587
  line L51 (-143.5774, -23.6368) -> (-143.5788, -22.8783)
  line L52 (-143.5788, -22.8783) -> (-143.3333, -22.8778)
  line L53 (-143.3333, -22.8778) -> (-143.3305, -24.3266)
  line L54 (-143.3305, -24.3266) -> (-143.5515, -24.3271)
  line L55 (-143.5515, -24.3271) -> (-143.552, -24.1074)
  spline S107 degree 3 poles (-143.552, -24.1074) (-143.5765, -24.1521) (-143.6182, -24.2281) (-143.6816, -24.2868) (-143.7078, -24.311) knots 0 0 0 0 0.015158 0.025781 0.025781 0.025781 0.025781
  spline S108 degree 3 poles (-143.7078, -24.311) (-143.7322, -24.3254) (-143.7808, -24.354) (-143.8372, -24.3583) (-143.8652, -24.3604) knots 0 0 0 0 0.008374 0.016702 0.016702 0.016702 0.016702
  spline S109 degree 3 poles (-143.8652, -24.3604) (-143.9078, -24.3566) (-143.9975, -24.3485) (-144.0763, -24.3047) (-144.1178, -24.2818) knots 0 0 0 0 0.012672 0.02671 0.02671 0.02671 0.02671
  line L56 (-144.1178, -24.2818) -> (-144.0336, -24.0538)
  spline S110 degree 3 poles (-144.0336, -24.0538) (-144.0042, -24.0692) (-143.9477, -24.099) (-143.884, -24.1041) (-143.8535, -24.1066) knots 0 0 0 0 0.009849 0.018951 0.018951 0.018951 0.018951
  spline S111 degree 3 poles (-143.8535, -24.1066) (-143.8273, -24.1046) (-143.7751, -24.1004) (-143.731, -24.0721) (-143.7089, -24.0579) knots 0 0 0 0 0.007735 0.015463 0.015463 0.015463 0.015463
  spline S112 degree 3 poles (-143.7089, -24.0579) (-143.689, -24.0398) (-143.6479, -24.0023) (-143.628, -23.9502) (-143.6178, -23.9234) knots 0 0 0 0 0.007973 0.016455 0.016455 0.016455 0.016455
  spline S113 degree 3 poles (-143.6178, -23.9234) (-143.6059, -23.8779) (-143.5815, -23.7839) (-143.5788, -23.6869) (-143.5774, -23.6368) knots 0 0 0 0 0.01405 0.029024 0.029024 0.029024 0.029024
  spline S114 degree 3 poles (-147.7392, -22.9196) (-147.6906, -22.9098) (-147.5842, -22.8883) (-147.4756, -22.8865) (-147.4167, -22.8856) knots 0 0 0 0 0.014862 0.032497 0.032497 0.032497 0.032497
  line L57 (-147.4167, -22.8856) -> (-146.654, -22.8841)
  line L58 (-146.654, -22.8841) -> (-146.6502, -24.8841)
  line L59 (-146.6502, -24.8841) -> (-147.4006, -24.8855)
  spline S115 degree 3 poles (-147.4006, -24.8855) (-147.4701, -24.8844) (-147.5958, -24.8823) (-147.715, -24.8431) (-147.7684, -24.8255) knots 0 0 0 0 0.020707 0.037453 0.037453 0.037453 0.037453
  spline S116 degree 3 poles (-147.7684, -24.8255) (-147.812, -24.8027) (-147.8989, -24.7574) (-147.9568, -24.6784) (-147.9856, -24.639) knots 0 0 0 0 0.014555 0.028975 0.028975 0.028975 0.028975
  spline S117 degree 3 poles (-147.9856, -24.639) (-148.0086, -24.597) (-148.0536, -24.5146) (-148.061, -24.421) (-148.0646, -24.3752) knots 0 0 0 0 0.014187 0.027818 0.027818 0.027818 0.027818
  spline S118 degree 3 poles (-148.0646, -24.3752) (-148.0616, -24.3329) (-148.0557, -24.2475) (-148.0157, -24.1718) (-147.9955, -24.1336) knots 0 0 0 0 0.01257 0.025379 0.025379 0.025379 0.025379
  spline S119 degree 3 poles (-147.9955, -24.1336) (-147.9684, -24.0972) (-147.9119, -24.021) (-147.829, -23.9746) (-147.7857, -23.9504) knots 0 0 0 0 0.013451 0.028132 0.028132 0.028132 0.028132
  spline S120 degree 3 poles (-147.7857, -23.9504) (-147.842, -23.9306) (-147.9498, -23.8927) (-148.0277, -23.8094) (-148.065, -23.7695) knots 0 0 0 0 0.017587 0.033722 0.033722 0.033722 0.033722
  spline S121 degree 3 poles (-148.065, -23.7695) (-148.0936, -23.7242) (-148.1519, -23.6318) (-148.1594, -23.5226) (-148.1632, -23.4668) knots 0 0 0 0 0.015782 0.032266 0.032266 0.032266 0.032266
  spline S122 degree 3 poles (-148.1632, -23.4668) (-148.1609, -23.421) (-148.1564, -23.3305) (-148.1215, -23.2468) (-148.1043, -23.2054) knots 0 0 0 0 0.013638 0.026971 0.026971 0.026971 0.026971
  spline S123 degree 3 poles (-148.1043, -23.2054) (-148.0843, -23.1681) (-148.0464, -23.0973) (-147.9864, -23.0441) (-147.958, -23.0189) knots 0 0 0 0 0.012583 0.02387 0.02387 0.02387 0.02387
  spline S124 degree 3 poles (-147.958, -23.0189) (-147.926, -22.9981) (-147.8581, -22.954) (-147.7803, -22.9315) (-147.7392, -22.9196) knots 0 0 0 0 0.011395 0.024144 0.024144 0.024144 0.024144
  spline S125 degree 3 poles (-150.4197, -23.1191) (-150.4315, -23.114) (-150.4581, -23.1023) (-150.4873, -23.1018) (-150.5037, -23.1015) knots 0 0 0 0 0.003804 0.008651 0.008651 0.008651 0.008651
  spline S126 degree 3 poles (-150.5037, -23.1015) (-150.5195, -23.1021) (-150.5556, -23.1035) (-150.5913, -23.1085) (-150.6114, -23.1113) knots 0 0 0 0 0.004747 0.010826 0.010826 0.010826 0.010826
  line L60 (-150.6114, -23.1113) -> (-150.6473, -22.8944)
  spline S127 degree 3 poles (-150.6473, -22.8944) (-150.6147, -22.888) (-150.5534, -22.8759) (-150.491, -22.8734) (-150.4618, -22.8722) knots 0 0 0 0 0.009958 0.018706 0.018706 0.018706 0.018706
  spline S128 degree 3 poles (-150.4618, -22.8722) (-150.4216, -22.8729) (-150.3497, -22.8742) (-150.2836, -22.9019) (-150.2544, -22.9141) knots 0 0 0 0 0.011916 0.021334 0.021334 0.021334 0.021334
  spline S129 degree 3 poles (-150.2544, -22.9141) (-150.2318, -22.9289) (-150.1881, -22.9575) (-150.1627, -23.0031) (-150.1505, -23.0251) knots 0 0 0 0 0.007959 0.015408 0.015408 0.015408 0.015408
  spline S130 degree 3 poles (-150.1505, -23.0251) (-150.1418, -23.0606) (-150.1185, -23.1556) (-150.1194, -23.2536) (-150.1199, -23.315) knots 0 0 0 0 0.010927 0.02924 0.02924 0.02924 0.02924
  line L61 (-150.1199, -23.315) -> (-150.1183, -24.1485)
  line L62 (-150.1183, -24.1485) -> (-149.9382, -24.1482)
  line L63 (-149.9382, -24.1482) -> (-149.9379, -24.3392)
  line L64 (-149.9379, -24.3392) -> (-150.118, -24.3395)
  line L65 (-150.118, -24.3395) -> (-150.1173, -24.6983)
  line L66 (-150.1173, -24.6983) -> (-150.3612, -24.8461)
  line L67 (-150.3612, -24.8461) -> (-150.3622, -24.34)
  line L68 (-150.3622, -24.34) -> (-150.6091, -24.3405)
  line L69 (-150.6091, -24.3405) -> (-150.6095, -24.1495)
  line L70 (-150.6095, -24.1495) -> (-150.3625, -24.149)
  line L71 (-150.3625, -24.149) -> (-150.3641, -23.3018)
  spline S131 degree 3 poles (-150.3641, -23.3018) (-150.3638, -23.2729) (-150.3633, -23.2273) (-150.3736, -23.183) (-150.3774, -23.1668) knots 0 0 0 0 0.008635 0.013608 0.013608 0.013608 0.013608
  spline S132 degree 3 poles (-150.3774, -23.1668) (-150.3824, -23.1572) (-150.3927, -23.138) (-150.4107, -23.1254) (-150.4197, -23.1191) knots 0 0 0 0 0.003189 0.00646 0.00646 0.00646 0.00646
  line L72 (-152.6719, -23.6541) -> (-152.6733, -22.8955)
  line L73 (-152.6733, -22.8955) -> (-152.4278, -22.8951)
  line L74 (-152.4278, -22.8951) -> (-152.425, -24.3439)
  line L75 (-152.425, -24.3439) -> (-152.646, -24.3443)
  line L76 (-152.646, -24.3443) -> (-152.6464, -24.1247)
  spline S133 degree 3 poles (-152.6464, -24.1247) (-152.671, -24.1694) (-152.7127, -24.2453) (-152.7761, -24.3041) (-152.8023, -24.3283) knots 0 0 0 0 0.015157 0.025781 0.025781 0.025781 0.025781
  spline S134 degree 3 poles (-152.8023, -24.3283) (-152.8267, -24.3426) (-152.8753, -24.3713) (-152.9317, -24.3755) (-152.9597, -24.3777) knots 0 0 0 0 0.008374 0.016702 0.016702 0.016702 0.016702
  spline S135 degree 3 poles (-152.9597, -24.3777) (-153.0023, -24.3738) (-153.092, -24.3657) (-153.1708, -24.322) (-153.2123, -24.299) knots 0 0 0 0 0.012672 0.02671 0.02671 0.02671 0.02671
  line L77 (-153.2123, -24.299) -> (-153.1281, -24.071)
  spline S136 degree 3 poles (-153.1281, -24.071) (-153.0987, -24.0865) (-153.0422, -24.1162) (-152.9785, -24.1214) (-152.948, -24.1239) knots 0 0 0 0 0.009849 0.018951 0.018951 0.018951 0.018951
  spline S137 degree 3 poles (-152.948, -24.1239) (-152.9218, -24.1218) (-152.8696, -24.1177) (-152.8255, -24.0894) (-152.8034, -24.0752) knots 0 0 0 0 0.007735 0.015463 0.015463 0.015463 0.015463
  spline S138 degree 3 poles (-152.8034, -24.0752) (-152.7835, -24.057) (-152.7424, -24.0195) (-152.7225, -23.9675) (-152.7123, -23.9406) knots 0 0 0 0 0.007973 0.016455 0.016455 0.016455 0.016455
  spline S139 degree 3 poles (-152.7123, -23.9406) (-152.7004, -23.8952) (-152.676, -23.8012) (-152.6733, -23.7041) (-152.6719, -23.6541) knots 0 0 0 0 0.01405 0.029024 0.029024 0.029024 0.029024
  line L78 (-153.9465, -24.9089) -> (-153.6471, -24.5263)
  line L79 (-153.6471, -24.5263) -> (-153.4438, -24.5259)
  line L80 (-153.4438, -24.5259) -> (-153.6246, -24.9083)
  line L81 (-153.6246, -24.9083) -> (-153.9465, -24.9089)
  circle A0 centre (-3, -3) radius 1.5
  circle A1 centre (-157, -27) radius 1.5
  circle A2 centre (-157, -77) radius 1.5
  line L82 (-155.4129, -22.9007) -> (-155.1564, -22.9003)
  spline S140 degree 3 poles (-155.1564, -22.9003) (-155.1447, -22.9275) (-155.1201, -22.9848) (-155.1114, -23.0465) (-155.1069, -23.0789) knots 0 0 0 0 0.008862 0.018609 0.018609 0.018609 0.018609
  spline S141 degree 3 poles (-155.1069, -23.0789) (-155.0637, -23.0437) (-154.983, -22.978) (-154.8885, -22.9347) (-154.8446, -22.9147) knots 0 0 0 0 0.016644 0.031058 0.031058 0.031058 0.031058
  spline S142 degree 3 poles (-154.8446, -22.9147) (-154.8014, -22.9007) (-154.7134, -22.8721) (-154.621, -22.8683) (-154.5739, -22.8664) knots 0 0 0 0 0.013561 0.027613 0.027613 0.027613 0.027613
  spline S143 degree 3 poles (-154.5739, -22.8664) (-154.5012, -22.8692) (-154.3676, -22.8743) (-154.2571, -22.9485) (-154.2067, -22.9824) knots 0 0 0 0 0.021312 0.039186 0.039186 0.039186 0.039186
  spline S144 degree 3 poles (-154.2067, -22.9824) (-154.1692, -23.0242) (-154.0933, -23.1091) (-154.0831, -23.2227) (-154.0779, -23.2802) knots 0 0 0 0 0.016401 0.033233 0.033233 0.033233 0.033233
  spline S145 degree 3 poles (-154.0779, -23.2802) (-154.0797, -23.3147) (-154.0833, -23.3826) (-154.1119, -23.4443) (-154.126, -23.4747) knots 0 0 0 0 0.010253 0.020199 0.020199 0.020199 0.020199
  spline S146 degree 3 poles (-154.126, -23.4747) (-154.1431, -23.5025) (-154.1769, -23.5572) (-154.2276, -23.5967) (-154.2526, -23.6161) knots 0 0 0 0 0.009704 0.019119 0.019119 0.019119 0.019119
  spline S147 degree 3 poles (-154.2526, -23.6161) (-154.2798, -23.6329) (-154.3353, -23.6671) (-154.3974, -23.6869) (-154.4291, -23.697) knots 0 0 0 0 0.009559 0.019479 0.019479 0.019479 0.019479
  spline S148 degree 3 poles (-154.4291, -23.697) (-154.4593, -23.7037) (-154.5313, -23.7197) (-154.6047, -23.7289) (-154.6473, -23.7342) knots 0 0 0 0 0.009264 0.022147 0.022147 0.022147 0.022147
  spline S149 degree 3 poles (-154.6473, -23.7342) (-154.7338, -23.7449) (-154.8819, -23.7631) (-155.0254, -23.803) (-155.0851, -23.8196) knots 0 0 0 0 0.02611 0.044656 0.044656 0.044656 0.044656
  spline S150 degree 3 poles (-155.0851, -23.8196) (-155.0854, -23.8334) (-155.086, -23.8548) (-155.0862, -23.8761) (-155.0863, -23.8838) knots 0 0 0 0 0.004128 0.006413 0.006413 0.006413 0.006413
  spline S151 degree 3 poles (-155.0863, -23.8838) (-155.0852, -23.9281) (-155.0834, -24.0064) (-155.0366, -24.0683) (-155.0163, -24.0951) knots 0 0 0 0 0.012908 0.022759 0.022759 0.022759 0.022759
  spline S152 degree 3 poles (-155.0163, -24.0951) (-154.9784, -24.1192) (-154.8935, -24.1732) (-154.7924, -24.1761) (-154.7365, -24.1778) knots 0 0 0 0 0.013259 0.029661 0.029661 0.029661 0.029661
  spline S153 degree 3 poles (-154.7365, -24.1778) (-154.6852, -24.1769) (-154.595, -24.1753) (-154.5152, -24.1343) (-154.4808, -24.1166) knots 0 0 0 0 0.015134 0.026599 0.026599 0.026599 0.026599
  spline S154 degree 3 poles (-154.4808, -24.1166) (-154.4546, -24.0899) (-154.3951, -24.0294) (-154.372, -23.9474) (-154.3591, -23.9015) knots 0 0 0 0 0.011056 0.025069 0.025069 0.025069 0.025069
  line L83 (-154.3591, -23.9015) -> (-154.119, -23.9338)
  spline S155 degree 3 poles (-154.119, -23.9338) (-154.1306, -23.9814) (-154.1523, -24.0707) (-154.2028, -24.1473) (-154.2263, -24.1829) knots 0 0 0 0 0.01459 0.02731 0.02731 0.02731 0.02731
  spline S156 degree 3 poles (-154.2263, -24.1829) (-154.2552, -24.2132) (-154.3168, -24.2775) (-154.3993, -24.3114) (-154.4429, -24.3293) knots 0 0 0 0 0.012433 0.026404 0.026404 0.026404 0.026404
  spline S157 degree 3 poles (-154.4429, -24.3293) (-154.4936, -24.3443) (-154.6008, -24.3761) (-154.7126, -24.3794) (-154.7716, -24.3811) knots 0 0 0 0 0.015787 0.033399 0.033399 0.033399 0.033399
  spline S158 degree 3 poles (-154.7716, -24.3811) (-154.8281, -24.3803) (-154.9305, -24.3787) (-155.029, -24.3506) (-155.0732, -24.338) knots 0 0 0 0 0.01685 0.030582 0.030582 0.030582 0.030582
  spline S159 degree 3 poles (-155.0732, -24.338) (-155.1082, -24.3239) (-155.1721, -24.298) (-155.2216, -24.2502) (-155.2439, -24.2285) knots 0 0 0 0 0.011204 0.020452 0.020452 0.020452 0.020452
  spline S160 degree 3 poles (-155.2439, -24.2285) (-155.2609, -24.2043) (-155.2967, -24.1534) (-155.3124, -24.0931) (-155.3206, -24.0616) knots 0 0 0 0 0.008807 0.018509 0.018509 0.018509 0.018509
  spline S161 degree 3 poles (-155.3206, -24.0616) (-155.3242, -24.0323) (-155.3334, -23.9571) (-155.3334, -23.8813) (-155.3333, -23.8351) knots 0 0 0 0 0.008847 0.022698 0.022698 0.022698 0.022698
  line L84 (-155.3333, -23.8351) -> (-155.334, -23.5077)
  spline S162 degree 3 poles (-155.334, -23.5077) (-155.3336, -23.4144) (-155.333, -23.2698) (-155.3459, -23.1257) (-155.3505, -23.0746) knots 0 0 0 0 0.027953 0.043363 0.043363 0.043363 0.043363
  spline S163 degree 3 poles (-155.3505, -23.0746) (-155.3571, -23.0445) (-155.3705, -22.9839) (-155.3987, -22.9286) (-155.4129, -22.9007) knots 0 0 0 0 0.009187 0.018535 0.018535 0.018535 0.018535
  line L85 (-153.702, -24.3463) -> (-153.7048, -22.8975)
  line L86 (-153.7048, -22.8975) -> (-153.4592, -22.897)
  line L87 (-153.4592, -22.897) -> (-153.4565, -24.3459)
  line L88 (-153.4565, -24.3459) -> (-153.702, -24.3463)
  spline S164 degree 3 poles (-151.4738, -23.0624) (-151.5166, -23.065) (-151.5993, -23.0701) (-151.67, -23.1131) (-151.7042, -23.1338) knots 0 0 0 0 0.012642 0.024448 0.024448 0.024448 0.024448
  spline S165 degree 3 poles (-151.7042, -23.1338) (-151.735, -23.163) (-151.8024, -23.2269) (-151.8366, -23.3135) (-151.8552, -23.3606) knots 0 0 0 0 0.012573 0.027537 0.027537 0.027537 0.027537
  line L89 (-151.8552, -23.3606) -> (-152.109, -23.3297)
  spline S166 degree 3 poles (-152.109, -23.3297) (-152.0858, -23.2604) (-152.041, -23.1263) (-151.9374, -23.0304) (-151.8873, -22.9841) knots 0 0 0 0 0.021523 0.041652 0.041652 0.041652 0.041652
  spline S167 degree 3 poles (-151.8873, -22.9841) (-151.8273, -22.9482) (-151.7, -22.872) (-151.5514, -22.8645) (-151.4728, -22.8605) knots 0 0 0 0 0.020652 0.043844 0.043844 0.043844 0.043844
  spline S168 degree 3 poles (-151.4728, -22.8605) (-151.3739, -22.8669) (-151.1848, -22.8791) (-151.0382, -22.9984) (-150.9683, -23.0553) knots 0 0 0 0 0.028913 0.055291 0.055291 0.055291 0.055291
  spline S169 degree 3 poles (-150.9683, -23.0553) (-150.914, -23.1309) (-150.7965, -23.2941) (-150.7865, -23.4958) (-150.7811, -23.6041) knots 0 0 0 0 0.027351 0.059089 0.059089 0.059089 0.059089
  spline S170 degree 3 poles (-150.7811, -23.6041) (-150.786, -23.716) (-150.7951, -23.9238) (-150.9136, -24.0936) (-150.9683, -24.172) knots 0 0 0 0 0.032809 0.060899 0.060899 0.060899 0.060899
  spline S171 degree 3 poles (-150.9683, -24.172) (-151.0367, -24.231) (-151.1769, -24.3519) (-151.3617, -24.3671) (-151.4563, -24.3748) knots 0 0 0 0 0.026399 0.05408 0.05408 0.05408 0.05408
  spline S172 degree 3 poles (-151.4563, -24.3748) (-151.5481, -24.3674) (-151.7279, -24.353) (-151.8645, -24.2355) (-151.9314, -24.1779) knots 0 0 0 0 0.026858 0.052633 0.052633 0.052633 0.052633
  spline S173 degree 3 poles (-151.9314, -24.1779) (-151.9852, -24.1013) (-152.1019, -23.9351) (-152.1115, -23.7314) (-152.1167, -23.6216) knots 0 0 0 0 0.027523 0.05971 0.05971 0.05971 0.05971
  spline S174 degree 3 poles (-152.1167, -23.6216) (-152.1166, -23.6125) (-152.1164, -23.5907) (-152.1158, -23.5689) (-152.1154, -23.5561) knots 0 0 0 0 0.002729 0.00655 0.00655 0.00655 0.00655
  line L90 (-152.1154, -23.5561) -> (-151.0349, -23.5541)
  spline S175 degree 3 poles (-151.0349, -23.5541) (-151.0422, -23.4814) (-151.0555, -23.3472) (-151.1345, -23.2385) (-151.1707, -23.1887) knots 0 0 0 0 0.021465 0.039604 0.039604 0.039604 0.039604
  spline S176 degree 3 poles (-151.1707, -23.1887) (-151.214, -23.1518) (-151.3014, -23.0773) (-151.416, -23.0674) (-151.4738, -23.0624) knots 0 0 0 0 0.016633 0.033577 0.033577 0.033577 0.033577
  line L91 (-149.7605, -22.89) -> (-149.504, -22.8895)
  spline S177 degree 3 poles (-149.504, -22.8895) (-149.4923, -22.9168) (-149.4677, -22.974) (-149.4591, -23.0358) (-149.4546, -23.0681) knots 0 0 0 0 0.008862 0.018609 0.018609 0.018609 0.018609
  spline S178 degree 3 poles (-149.4546, -23.0681) (-149.4113, -23.0329) (-149.3307, -22.9673) (-149.2361, -22.924) (-149.1923, -22.9039) knots 0 0 0 0 0.016644 0.031058 0.031058 0.031058 0.031058
  spline S179 degree 3 poles (-149.1923, -22.9039) (-149.149, -22.8899) (-149.061, -22.8614) (-148.9686, -22.8576) (-148.9215, -22.8557) knots 0 0 0 0 0.013561 0.027613 0.027613 0.027613 0.027613
  spline S180 degree 3 poles (-148.9215, -22.8557) (-148.8489, -22.8584) (-148.7153, -22.8635) (-148.6047, -22.9378) (-148.5543, -22.9716) knots 0 0 0 0 0.021312 0.039186 0.039186 0.039186 0.039186
  spline S181 degree 3 poles (-148.5543, -22.9716) (-148.5169, -23.0135) (-148.4409, -23.0984) (-148.4307, -23.212) (-148.4255, -23.2695) knots 0 0 0 0 0.016401 0.033233 0.033233 0.033233 0.033233